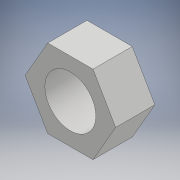
# Autodesk Inventor part: M5 Nut
Saved by Autodesk Inventor 2017 (Build 210142000, 142)
## iProperties
Created: 2017-03-29
Part Number: M5 Nut
Material: Generic
Document SubType Name: Modeling
Designer: umr
Density: 1 g/cm^3
Appearance: Default
Author: umr
Autodesk Inventor part; units mm, degrees
ref_plane "YZ Plane" through (0, 0, 0) normal (1, 0, 0) x (0, 1, 0)
ref_plane "XZ Plane" through (0, 0, 0) normal (0, 1, 0) x (-1, 0, 0)
ref_plane "XY Plane" through (0, 0, 0) normal (0, 0, 1) x (1, 0, 0)
sketch "Sketch1" plane through (0, 0, 0) normal (0, 1, 0) x (-1, 0, 0)
  line L0 (-4.4381, 0) -> (-2.219, 3.8435)
  line L1 (-2.219, 3.8435) -> (2.219, 3.8435)
  line L2 (2.219, 3.8435) -> (4.4381, 0)
  line L3 (4.4381, 0) -> (2.219, -3.8435)
  line L4 (2.219, -3.8435) -> (-2.219, -3.8435)
  line L5 (-2.219, -3.8435) -> (-4.4381, 0)
  circle A0 centre (0, 0) radius 2.5
  dimension "d0" = 7.687
  dimension "d1" = 5
  constraints: 12 end point, 2 coincident, 1 centre point, 13 other
  measures "d0" distance between parallel lines of L4 L1
  measures "d1" diameter of A0
extrude "Extrusion1" add sketch "Sketch1" along normal blind 3.85
body "Solid1"
